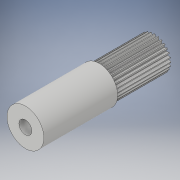
# Autodesk Inventor part: Part10
Saved by Autodesk Inventor 2017 SP1 (Build 210196100, 196)
## iProperties
Created: 2017-05-14
Part Number: Part10
Material: Generic
Document SubType Name: Modeling
Designer: Zach
Density: 1 g/cm^3
Appearance: Default
Author: Zach
Autodesk Inventor part; units mm, degrees
ref_plane "YZ Plane" through (0, 0, 0) normal (1, 0, 0) x (0, 1, 0)
ref_plane "XZ Plane" through (0, 0, 0) normal (0, 1, 0) x (-1, 0, 0)
ref_plane "XY Plane" through (0, 0, 0) normal (0, 0, 1) x (1, 0, 0)
sketch "Sketch1" plane through (0, 0, 0) normal (0, 0, 1) x (1, 0, 0)
  circle A0 centre (0, 0) radius 10
  dimension "d0" = 20
  constraints: 1 centre point, 1 coincident
  measures "d0" diameter of A0
extrude "Extrusion1" add sketch "Sketch1" along normal blind 40
sketch "Sketch2" plane through (0, 0, 0) normal (0, 0, -1) x (-1, 0, 0)
  circle A0 centre (0, 0) radius 7.5
  dimension "d3" = 15
  constraints: 1 centre point, 1 coincident
  measures "d3" diameter of A0
extrude "Extrusion2" add sketch "Sketch2" along normal blind 30
sketch "Sketch3" plane through (0, 0, -30) normal (0, 0, -1) x (-1, 0, 0)
  circle A0 centre (0, 0) radius 3.5
  dimension "d6" = 7
  constraints: 1 centre point, 1 coincident
  measures "d6" diameter of A0
extrude "Extrusion3" cut sketch "Sketch3" against normal through all
sketch "Sketch4" plane through (0, 0, 0) normal (0, 0, -1) x (-1, 0, 0)
  line L0 (0, 0) -> (0, 11.2895) construction
  arc A0 (0.7, 7.4673) -> (-0.7, 7.4673) centre (0, 0) ccw
  line L1 (-0.7, 7.4673) -> (0, 9.5) construction
  line L2 (0.7, 7.4673) -> (0, 9.5) construction
  line L3 (-0.7, 7.4673) -> (-0.2116, 8.8855)
  line L4 (-0.2116, 8.8855) -> (0.2116, 8.8855)
  line L5 (0.7, 7.4673) -> (0.2116, 8.8855)
  arc A1 (-0.9792, 7.4358) -> (-2.3441, 7.1243) centre (0, 0) ccw
  line L6 (-2.1835, 8.6157) -> (-1.7709, 8.7098)
  line L7 (-2.3441, 7.1243) -> (-2.1139, 9.2618) construction
  line L8 (-2.3441, 7.1243) -> (-2.1835, 8.6157)
  line L9 (-0.9792, 7.4358) -> (-2.1139, 9.2618) construction
  line L10 (-0.9792, 7.4358) -> (-1.7709, 8.7098)
  arc A2 (-2.6092, 7.0315) -> (-3.8706, 6.4241) centre (0, 0) ccw
  line L11 (-4.0459, 7.9138) -> (-3.6646, 8.0974)
  line L12 (-3.8706, 6.4241) -> (-4.1219, 8.5592) construction
  line L13 (-3.8706, 6.4241) -> (-4.0459, 7.9138)
  line L14 (-2.6092, 7.0315) -> (-4.1219, 8.5592) construction
  line L15 (-2.6092, 7.0315) -> (-3.6646, 8.0974)
  arc A3 (-4.1085, 6.2746) -> (-5.203, 5.4017) centre (0, 0) ccw
  line L16 (-5.7055, 6.8151) -> (-5.3746, 7.0789)
  line L17 (-5.203, 5.4017) -> (-5.9232, 7.4274) construction
  line L18 (-5.203, 5.4017) -> (-5.7055, 6.8151)
  line L19 (-4.1085, 6.2746) -> (-5.9232, 7.4274) construction
  line L20 (-4.1085, 6.2746) -> (-5.3746, 7.0789)
  arc A4 (-5.4017, 5.203) -> (-6.2746, 4.1085) centre (0, 0) ccw
  line L21 (-7.0789, 5.3746) -> (-6.8151, 5.7055)
  line L22 (-6.2746, 4.1085) -> (-7.4274, 5.9232) construction
  line L23 (-6.2746, 4.1085) -> (-7.0789, 5.3746)
  line L24 (-5.4017, 5.203) -> (-7.4274, 5.9232) construction
  line L25 (-5.4017, 5.203) -> (-6.8151, 5.7055)
  arc A5 (-6.4241, 3.8706) -> (-7.0315, 2.6092) centre (0, 0) ccw
  line L26 (-8.0974, 3.6646) -> (-7.9138, 4.0459)
  line L27 (-7.0315, 2.6092) -> (-8.5592, 4.1219) construction
  line L28 (-7.0315, 2.6092) -> (-8.0974, 3.6646)
  line L29 (-6.4241, 3.8706) -> (-8.5592, 4.1219) construction
  line L30 (-6.4241, 3.8706) -> (-7.9138, 4.0459)
  arc A6 (-7.1243, 2.3441) -> (-7.4358, 0.9792) centre (0, 0) ccw
  line L31 (-8.7098, 1.7709) -> (-8.6157, 2.1835)
  line L32 (-7.4358, 0.9792) -> (-9.2618, 2.1139) construction
  line L33 (-7.4358, 0.9792) -> (-8.7098, 1.7709)
  line L34 (-7.1243, 2.3441) -> (-9.2618, 2.1139) construction
  line L35 (-7.1243, 2.3441) -> (-8.6157, 2.1835)
  arc A7 (-7.4673, 0.7) -> (-7.4673, -0.7) centre (0, 0) ccw
  line L36 (-8.8855, -0.2116) -> (-8.8855, 0.2116)
  line L37 (-7.4673, -0.7) -> (-9.5, 0) construction
  line L38 (-7.4673, -0.7) -> (-8.8855, -0.2116)
  line L39 (-7.4673, 0.7) -> (-9.5, 0) construction
  line L40 (-7.4673, 0.7) -> (-8.8855, 0.2116)
  arc A8 (-7.4358, -0.9792) -> (-7.1243, -2.3441) centre (0, 0) ccw
  line L41 (-8.6157, -2.1835) -> (-8.7098, -1.7709)
  line L42 (-7.1243, -2.3441) -> (-9.2618, -2.1139) construction
  line L43 (-7.1243, -2.3441) -> (-8.6157, -2.1835)
  line L44 (-7.4358, -0.9792) -> (-9.2618, -2.1139) construction
  line L45 (-7.4358, -0.9792) -> (-8.7098, -1.7709)
  arc A9 (-7.0315, -2.6092) -> (-6.4241, -3.8706) centre (0, 0) ccw
  line L46 (-7.9138, -4.0459) -> (-8.0974, -3.6646)
  line L47 (-6.4241, -3.8706) -> (-8.5592, -4.1219) construction
  line L48 (-6.4241, -3.8706) -> (-7.9138, -4.0459)
  line L49 (-7.0315, -2.6092) -> (-8.5592, -4.1219) construction
  line L50 (-7.0315, -2.6092) -> (-8.0974, -3.6646)
  arc A10 (-6.2746, -4.1085) -> (-5.4017, -5.203) centre (0, 0) ccw
  line L51 (-6.8151, -5.7055) -> (-7.0789, -5.3746)
  line L52 (-5.4017, -5.203) -> (-7.4274, -5.9232) construction
  line L53 (-5.4017, -5.203) -> (-6.8151, -5.7055)
  line L54 (-6.2746, -4.1085) -> (-7.4274, -5.9232) construction
  line L55 (-6.2746, -4.1085) -> (-7.0789, -5.3746)
  arc A11 (-5.203, -5.4017) -> (-4.1085, -6.2746) centre (0, 0) ccw
  line L56 (-5.3746, -7.0789) -> (-5.7055, -6.8151)
  line L57 (-4.1085, -6.2746) -> (-5.9232, -7.4274) construction
  line L58 (-4.1085, -6.2746) -> (-5.3746, -7.0789)
  line L59 (-5.203, -5.4017) -> (-5.9232, -7.4274) construction
  line L60 (-5.203, -5.4017) -> (-5.7055, -6.8151)
  arc A12 (-3.8706, -6.4241) -> (-2.6092, -7.0315) centre (0, 0) ccw
  line L61 (-3.6646, -8.0974) -> (-4.0459, -7.9138)
  line L62 (-2.6092, -7.0315) -> (-4.1219, -8.5592) construction
  line L63 (-2.6092, -7.0315) -> (-3.6646, -8.0974)
  line L64 (-3.8706, -6.4241) -> (-4.1219, -8.5592) construction
  line L65 (-3.8706, -6.4241) -> (-4.0459, -7.9138)
  arc A13 (-2.3441, -7.1243) -> (-0.9792, -7.4358) centre (0, 0) ccw
  line L66 (-1.7709, -8.7098) -> (-2.1835, -8.6157)
  line L67 (-0.9792, -7.4358) -> (-2.1139, -9.2618) construction
  line L68 (-0.9792, -7.4358) -> (-1.7709, -8.7098)
  line L69 (-2.3441, -7.1243) -> (-2.1139, -9.2618) construction
  line L70 (-2.3441, -7.1243) -> (-2.1835, -8.6157)
  arc A14 (-0.7, -7.4673) -> (0.7, -7.4673) centre (0, 0) ccw
  line L71 (0.2116, -8.8855) -> (-0.2116, -8.8855)
  line L72 (0.7, -7.4673) -> (0, -9.5) construction
  line L73 (0.7, -7.4673) -> (0.2116, -8.8855)
  line L74 (-0.7, -7.4673) -> (0, -9.5) construction
  line L75 (-0.7, -7.4673) -> (-0.2116, -8.8855)
  arc A15 (0.9792, -7.4358) -> (2.3441, -7.1243) centre (0, 0) ccw
  line L76 (2.1835, -8.6157) -> (1.7709, -8.7098)
  line L77 (2.3441, -7.1243) -> (2.1139, -9.2618) construction
  line L78 (2.3441, -7.1243) -> (2.1835, -8.6157)
  line L79 (0.9792, -7.4358) -> (2.1139, -9.2618) construction
  line L80 (0.9792, -7.4358) -> (1.7709, -8.7098)
  arc A16 (2.6092, -7.0315) -> (3.8706, -6.4241) centre (0, 0) ccw
  line L81 (4.0459, -7.9138) -> (3.6646, -8.0974)
  line L82 (3.8706, -6.4241) -> (4.1219, -8.5592) construction
  line L83 (3.8706, -6.4241) -> (4.0459, -7.9138)
  line L84 (2.6092, -7.0315) -> (4.1219, -8.5592) construction
  line L85 (2.6092, -7.0315) -> (3.6646, -8.0974)
  arc A17 (4.1085, -6.2746) -> (5.203, -5.4017) centre (0, 0) ccw
  line L86 (5.7055, -6.8151) -> (5.3746, -7.0789)
  line L87 (5.203, -5.4017) -> (5.9232, -7.4274) construction
  line L88 (5.203, -5.4017) -> (5.7055, -6.8151)
  line L89 (4.1085, -6.2746) -> (5.9232, -7.4274) construction
  line L90 (4.1085, -6.2746) -> (5.3746, -7.0789)
  arc A18 (5.4017, -5.203) -> (6.2746, -4.1085) centre (0, 0) ccw
  line L91 (7.0789, -5.3746) -> (6.8151, -5.7055)
  line L92 (6.2746, -4.1085) -> (7.4274, -5.9232) construction
  line L93 (6.2746, -4.1085) -> (7.0789, -5.3746)
  line L94 (5.4017, -5.203) -> (7.4274, -5.9232) construction
  line L95 (5.4017, -5.203) -> (6.8151, -5.7055)
  arc A19 (6.4241, -3.8706) -> (7.0315, -2.6092) centre (0, 0) ccw
  line L96 (8.0974, -3.6646) -> (7.9138, -4.0459)
  line L97 (7.0315, -2.6092) -> (8.5592, -4.1219) construction
  line L98 (7.0315, -2.6092) -> (8.0974, -3.6646)
  line L99 (6.4241, -3.8706) -> (8.5592, -4.1219) construction
  line L100 (6.4241, -3.8706) -> (7.9138, -4.0459)
  arc A20 (7.1243, -2.3441) -> (7.4358, -0.9792) centre (0, 0) ccw
  line L101 (8.7098, -1.7709) -> (8.6157, -2.1835)
  line L102 (7.4358, -0.9792) -> (9.2618, -2.1139) construction
  line L103 (7.4358, -0.9792) -> (8.7098, -1.7709)
  line L104 (7.1243, -2.3441) -> (9.2618, -2.1139) construction
  line L105 (7.1243, -2.3441) -> (8.6157, -2.1835)
  arc A21 (7.4673, -0.7) -> (7.4673, 0.7) centre (0, 0) ccw
  line L106 (8.8855, 0.2116) -> (8.8855, -0.2116)
  line L107 (7.4673, 0.7) -> (9.5, 0) construction
  line L108 (7.4673, 0.7) -> (8.8855, 0.2116)
  line L109 (7.4673, -0.7) -> (9.5, 0) construction
  line L110 (7.4673, -0.7) -> (8.8855, -0.2116)
  arc A22 (7.4358, 0.9792) -> (7.1243, 2.3441) centre (0, 0) ccw
  line L111 (8.6157, 2.1835) -> (8.7098, 1.7709)
  line L112 (7.1243, 2.3441) -> (9.2618, 2.1139) construction
  line L113 (7.1243, 2.3441) -> (8.6157, 2.1835)
  line L114 (7.4358, 0.9792) -> (9.2618, 2.1139) construction
  line L115 (7.4358, 0.9792) -> (8.7098, 1.7709)
  arc A23 (7.0315, 2.6092) -> (6.4241, 3.8706) centre (0, 0) ccw
  line L116 (7.9138, 4.0459) -> (8.0974, 3.6646)
  line L117 (6.4241, 3.8706) -> (8.5592, 4.1219) construction
  line L118 (6.4241, 3.8706) -> (7.9138, 4.0459)
  line L119 (7.0315, 2.6092) -> (8.5592, 4.1219) construction
  line L120 (7.0315, 2.6092) -> (8.0974, 3.6646)
  arc A24 (6.2746, 4.1085) -> (5.4017, 5.203) centre (0, 0) ccw
  line L121 (6.8151, 5.7055) -> (7.0789, 5.3746)
  line L122 (5.4017, 5.203) -> (7.4274, 5.9232) construction
  line L123 (5.4017, 5.203) -> (6.8151, 5.7055)
  line L124 (6.2746, 4.1085) -> (7.4274, 5.9232) construction
  line L125 (6.2746, 4.1085) -> (7.0789, 5.3746)
  arc A25 (5.203, 5.4017) -> (4.1085, 6.2746) centre (0, 0) ccw
  line L126 (5.3746, 7.0789) -> (5.7055, 6.8151)
  line L127 (4.1085, 6.2746) -> (5.9232, 7.4274) construction
  line L128 (4.1085, 6.2746) -> (5.3746, 7.0789)
  line L129 (5.203, 5.4017) -> (5.9232, 7.4274) construction
  line L130 (5.203, 5.4017) -> (5.7055, 6.8151)
  arc A26 (3.8706, 6.4241) -> (2.6092, 7.0315) centre (0, 0) ccw
  line L131 (3.6646, 8.0974) -> (4.0459, 7.9138)
  line L132 (2.6092, 7.0315) -> (4.1219, 8.5592) construction
  line L133 (2.6092, 7.0315) -> (3.6646, 8.0974)
  line L134 (3.8706, 6.4241) -> (4.1219, 8.5592) construction
  line L135 (3.8706, 6.4241) -> (4.0459, 7.9138)
  arc A27 (2.3441, 7.1243) -> (0.9792, 7.4358) centre (0, 0) ccw
  line L136 (1.7709, 8.7098) -> (2.1835, 8.6157)
  line L137 (0.9792, 7.4358) -> (2.1139, 9.2618) construction
  line L138 (0.9792, 7.4358) -> (1.7709, 8.7098)
  line L139 (2.3441, 7.1243) -> (2.1139, 9.2618) construction
  line L140 (2.3441, 7.1243) -> (2.1835, 8.6157)
  circle A28 centre (0, 0) radius 7.5 projected
  dimension "d9" = 9.5
  dimension "d12" = 7.5
  dimension "d19" = 1.5
  dimension "d21" = 1.4
  dimension "d24" = 360
  constraints: 282 end point, 57 point on line, 56 point on circle, 28 centre point, 2 coincident, 1 collinear, 1 concentric, 1 horizontal, 1 symmetric about line, 1 vertical, 335 other
  measures "d9" distance of L0.start L1.end
  measures "d12" radius of A0
  measures "d19" distance of L1.start L3.end
  measures "d21" distance of L2.start L1.start
extrude "Extrusion4" add sketch "Sketch4" along normal blind 30 contours A0 L3 L4 L5 | L138 L136 L140 A27 | A1 L8 L6 L10 | L133 L131 L135 A26 | A2 L13 L11 L15 | L128 L126 L130 A25 | A3 L18 L16 L20 | L123 L121 L125 A24 | A4 L23 L21 L25 | L118 L116 L120 A23 | A5 L28 L26 L30 | L113 L111 L115 A22 | A6 L33 L31 L35 | L108 L106 L110 A21 | A7 L38 L36 L40 | A8 L43 L41 L45 | L103 L101 L105 A20 | A9 L48 L46 L50 | L98 L96 L100 A19 | A10 L53 L51 L55 | L93 L91 L95 A18 | A11 L58 L56 L60 | L88 L86 L90 A17 | A12 L63 L61 L65 | L83 L81 L85 A16 | A13 L68 L66 L70 | L78 L76 L80 A15 | A14 L73 L71 L75
body "Solid1"
